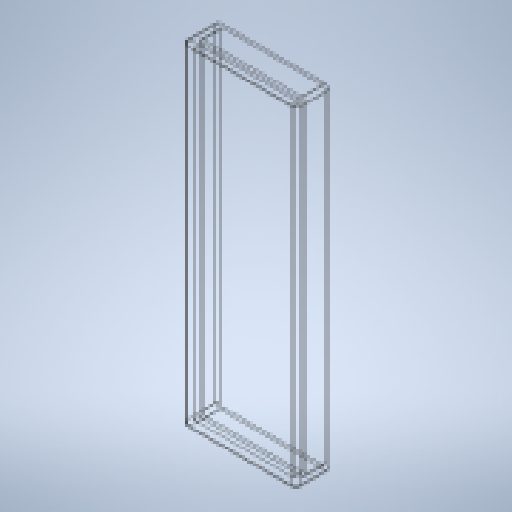
# Autodesk Inventor part: Tapa bateria
Saved by Autodesk Inventor 2024.2 (Build 282272000, 272)
## iProperties
Created: 2024-12-01
Part Number: Tapa bateria
Material: Genérico
Document SubType Name: Modeling
Designer: sergi
Density: 1 g/cm^3
Appearance: Valor por defecto
Author: sergi
Autodesk Inventor part; units mm, degrees
ref_plane "YZ Plane" through (0, 0, 0) normal (1, 0, 0) x (0, 1, 0)
ref_plane "XZ Plane" through (0, 0, 0) normal (0, 1, 0) x (-1, 0, 0)
ref_plane "XY Plane" through (0, 0, 0) normal (0, 0, 1) x (1, 0, 0)
sketch "Boceto1" plane through (0, 0, 0) normal (0, 0, 1) x (1, 0, 0)
  line L0 (-22.25, 73.85) -> (22.25, 73.85) projected
  line L1 (23.85, 72.25) -> (23.85, -72.25) projected
  line L2 (22.25, -73.85) -> (-22.25, -73.85) projected
  line L3 (-23.85, -72.25) -> (-23.85, 72.25) projected
  line L4 (23.65, -75.25) -> (-23.65, -75.25) projected
  line L5 (25.25, 73.65) -> (25.25, -73.65) projected
  line L6 (-23.65, 75.25) -> (23.65, 75.25) projected
  line L7 (-25.25, -73.65) -> (-25.25, 73.65) projected
  line L8 (-22.25, 72.25) -> (22.25, 72.25) projected
  line L9 (-22.25, -72.25) -> (-22.25, 72.25) projected
  line L10 (22.25, 72.25) -> (22.25, -72.25) projected
  line L11 (22.25, -72.25) -> (-22.25, -72.25) projected
  line L12 (25.45, 75.45) -> (-25.45, 75.45)
  line L13 (-25.45, 75.45) -> (-25.45, -75.45)
  line L14 (-25.45, -75.45) -> (25.45, -75.45)
  line L15 (25.45, -75.45) -> (25.45, 75.45)
  arc A0 (23.85, 72.25) -> (22.25, 73.85) centre (22.25, 72.25) ccw projected
  arc A1 (22.25, -73.85) -> (23.85, -72.25) centre (22.25, -72.25) ccw projected
  arc A2 (-23.85, -72.25) -> (-22.25, -73.85) centre (-22.25, -72.25) ccw projected
  arc A3 (-22.25, 73.85) -> (-23.85, 72.25) centre (-22.25, 72.25) ccw projected
  arc A4 (23.65, -75.25) -> (25.25, -73.65) centre (23.65, -73.65) ccw projected
  arc A5 (25.25, 73.65) -> (23.65, 75.25) centre (23.65, 73.65) ccw projected
  arc A6 (-23.65, 75.25) -> (-25.25, 73.65) centre (-23.65, 73.65) ccw projected
  arc A7 (-25.25, -73.65) -> (-23.65, -75.25) centre (-23.65, -73.65) ccw projected
  line L16 (-22.25, -74.05) -> (22.25, -74.05)
  arc A8 (22.25, -74.05) -> (24.05, -72.25) centre (22.25, -72.25) ccw
  line L17 (24.05, -72.25) -> (24.05, 72.25)
  arc A9 (24.05, 72.25) -> (22.25, 74.05) centre (22.25, 72.25) ccw
  line L18 (22.25, 74.05) -> (-22.25, 74.05)
  arc A10 (-22.25, 74.05) -> (-24.05, 72.25) centre (-22.25, 72.25) ccw
  line L19 (-24.05, 72.25) -> (-24.05, -72.25)
  arc A11 (-24.05, -72.25) -> (-22.25, -74.05) centre (-22.25, -72.25) ccw
  point P0 (0, 0)
  dimension "d0" = 1.6
  dimension "d10" = 0.2
  constraints: 16 end point, 8 point on circle, 4 centre point, 10 other
  measures "d0" distance between parallel lines of L0 L12
  measures "d10" distance between parallel lines of L2 L16
extrude "Extrusión1" add sketch "Boceto1" along normal blind 9 contours L4 A7 L7 A6 L6 A5 L5 A4 | L15 L14 L13 L12
sketch "Boceto2" plane through (0, 0, 9) normal (0, 0, 1) x (1, 0, 0)
  line L0 (-25.45, 75.45) -> (-25.45, -75.45) construction
  line L1 (-25.45, -75.45) -> (25.45, -75.45) construction
  line L2 (25.45, -75.45) -> (25.45, 75.45) construction
  line L3 (25.45, 75.45) -> (-25.45, 75.45) construction
  line L4 (-22.45, 72.45) -> (-22.45, -72.45)
  line L5 (-22.45, -72.45) -> (22.45, -72.45)
  line L6 (22.45, -72.45) -> (22.45, 72.45)
  line L7 (22.45, 72.45) -> (-22.45, 72.45)
  line L8 (-25.45, 75.45) -> (-25.45, -75.45)
  line L9 (-25.45, -75.45) -> (25.45, -75.45)
  line L10 (25.45, -75.45) -> (25.45, 75.45)
  line L11 (25.45, 75.45) -> (-25.45, 75.45)
  point P0 (0, 0)
  dimension "d3" = 3
  dimension "d4" = 3
  constraints: 16 end point, 6 other
  measures "d3" distance between parallel lines of L3 L7
  measures "d4" distance between parallel lines of L7 L11
extrude "Extrusión2" add sketch "Boceto2" along normal blind 4
sketch "Boceto3" plane through (0, 0, 13) normal (0, 0, 1) x (1, 0, 0)
  line L0 (-25.45, -75.45) -> (25.45, -75.45) projected
  line L1 (25.45, -75.45) -> (25.45, 75.45) projected
  line L2 (25.45, 75.45) -> (-25.45, 75.45) projected
  line L3 (-25.45, 75.45) -> (-25.45, -75.45) projected
  line L4 (-22.45, 72.45) -> (22.45, 72.45) projected
  line L5 (22.45, 72.45) -> (22.45, -72.45) projected
  line L6 (22.45, -72.45) -> (-22.45, -72.45) projected
  line L7 (-22.45, -72.45) -> (-22.45, 72.45) projected
  point P0 (0, 0)
extrude "Extrusión3" add sketch "Boceto3" along normal blind 2 contours L3 L2 L1 L0 | L4 L5 L6 L7
fillet "Empalme1" radius 1.6 11 edges at (25.45, -75.45, 12) (25.45, -75.45, 4.5) (-25.45, -75.45, 12) (-25.45, -75.45, 4.5) (-25.45, 75.45, 7.5) (25.45, 75.45, 12) (25.45, 75.45, 4.5) (25.45, 0, 15) (0, 75.45, 15) (-25.45, 0, 15) (0, -75.45, 15)
